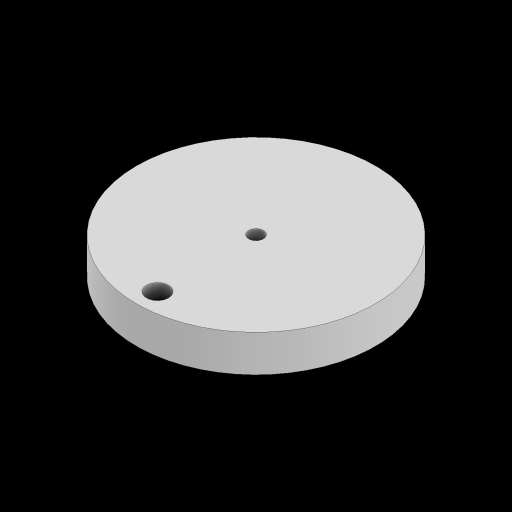
# Autodesk Inventor part: SC-1-02-Circle Arc Cover
Saved by Autodesk Inventor 2023 (Build 270158000, 158)
## iProperties
Created: 2022-12-08
Part Number: SC-1-02-Circle Arc Cover
Material: Generic
Document SubType Name: Modeling
Designer: annah
Density: 1 g/cm^3
Appearance: Default
Author: annah
Autodesk Inventor part; units mm, degrees
ref_plane "YZ Plane" through (0, 0, 0) normal (1, 0, 0) x (0, 1, 0)
ref_plane "XZ Plane" through (0, 0, 0) normal (0, 1, 0) x (-1, 0, 0)
ref_plane "XY Plane" through (0, 0, 0) normal (0, 0, 1) x (1, 0, 0)
sketch "Sketch1" plane through (0, 0, 0) normal (0, 1, 0) x (-1, 0, 0)
  line L0 (0, 0) -> (18.5658, -69.2885)
  circle A0 centre (25.8819, -96.5926) radius 5
  arc A1 (24.729, -72.9816) -> (15.0747, -75.5678) centre (19.8599, -74.1181) ccw
  line L1 (30.6777, -95.1782) -> (24.6448, -72.6673)
  line L2 (21.0523, -97.8867) -> (14.9907, -75.2542)
  circle A2 centre (0, -103.5276) radius 11.6229
  line L3 (21.0523, -97.8867) -> (25.8819, -96.5926)
  arc A3 (-25.8819, -96.5926) -> (26.7197, -101.5219) centre (0, -103.5276) ccw
  circle A4 centre (0, -103.5276) radius 39.9
  arc A5 (57.9067, -50.8394) -> (50.8389, -57.9063) centre (54.2582, -54.2582) ccw
  line L4 (67.1751, -74.2462) -> (50.6094, -57.6767)
  line L5 (74.1567, -67.0879) -> (57.6767, -50.6094)
  circle A6 centre (70.7107, -70.7107) radius 5
  circle A7 centre (51.7638, -89.6575) radius 11.6229
  arc A8 (75.5684, -15.0748) -> (72.9809, -24.7289) centre (74.1181, -19.8599) ccw
  line L6 (95.2985, -30.7115) -> (72.6673, -24.6448)
  line L7 (97.7655, -21.0214) -> (75.2542, -14.9907)
  circle A9 centre (96.5926, -25.8819) radius 5
  circle A10 centre (89.6575, -51.7638) radius 11.6229
  arc A11 (72.9816, 24.729) -> (75.5678, 15.0747) centre (74.1181, 19.8599) ccw
  line L8 (97.8867, 21.0523) -> (75.2542, 14.9907)
  line L9 (95.1782, 30.6777) -> (72.6673, 24.6448)
  circle A12 centre (96.5926, 25.8819) radius 5
  circle A13 centre (103.5276, 0) radius 11.6229
  arc A14 (50.8394, 57.9067) -> (57.9063, 50.8389) centre (54.2582, 54.2582) ccw
  line L10 (74.2462, 67.1751) -> (57.6767, 50.6094)
  line L11 (67.0879, 74.1567) -> (50.6094, 57.6767)
  circle A15 centre (70.7107, 70.7107) radius 5
  circle A16 centre (89.6575, 51.7638) radius 11.6229
  arc A17 (15.0748, 75.5684) -> (24.7289, 72.9809) centre (19.8599, 74.1181) ccw
  line L12 (30.7115, 95.2985) -> (24.6448, 72.6673)
  line L13 (21.0214, 97.7655) -> (14.9907, 75.2542)
  circle A18 centre (25.8819, 96.5926) radius 5
  circle A19 centre (51.7638, 89.6575) radius 11.6229
  arc A20 (-24.729, 72.9816) -> (-15.0747, 75.5678) centre (-19.8599, 74.1181) ccw
  line L14 (-21.0523, 97.8867) -> (-14.9907, 75.2542)
  line L15 (-30.6777, 95.1782) -> (-24.6448, 72.6673)
  circle A21 centre (-25.8819, 96.5926) radius 5
  circle A22 centre (0, 103.5276) radius 11.6229
  arc A23 (-57.9067, 50.8394) -> (-50.8389, 57.9063) centre (-54.2582, 54.2582) ccw
  line L16 (-67.1751, 74.2462) -> (-50.6094, 57.6767)
  line L17 (-74.1567, 67.0879) -> (-57.6767, 50.6094)
  circle A24 centre (-70.7107, 70.7107) radius 5
  circle A25 centre (-51.7638, 89.6575) radius 11.6229
  arc A26 (-75.5684, 15.0748) -> (-72.9809, 24.7289) centre (-74.1181, 19.8599) ccw
  line L18 (-95.2985, 30.7115) -> (-72.6673, 24.6448)
  line L19 (-97.7655, 21.0214) -> (-75.2542, 14.9907)
  circle A27 centre (-96.5926, 25.8819) radius 5
  circle A28 centre (-89.6575, 51.7638) radius 11.6229
  arc A29 (-72.9816, -24.729) -> (-75.5678, -15.0747) centre (-74.1181, -19.8599) ccw
  line L20 (-97.8867, -21.0523) -> (-75.2542, -14.9907)
  line L21 (-95.1782, -30.6777) -> (-72.6673, -24.6448)
  circle A30 centre (-96.5926, -25.8819) radius 5
  circle A31 centre (-103.5276, 0) radius 11.6229
  arc A32 (-50.8394, -57.9067) -> (-57.9063, -50.8389) centre (-54.2582, -54.2582) ccw
  line L22 (-74.2462, -67.1751) -> (-57.6767, -50.6094)
  line L23 (-67.0879, -74.1567) -> (-50.6094, -57.6767)
  circle A33 centre (-70.7107, -70.7107) radius 5
  circle A34 centre (-89.6575, -51.7638) radius 11.6229
  arc A35 (-15.0748, -75.5684) -> (-24.7289, -72.9809) centre (-19.8599, -74.1181) ccw
  line L24 (-30.7115, -95.2985) -> (-24.6448, -72.6673)
  line L25 (-21.0214, -97.7655) -> (-14.9907, -75.2542)
  circle A36 centre (-25.8819, -96.5926) radius 5
  circle A37 centre (-51.7638, -89.6575) radius 11.6229
  circle A38 centre (0, 0) radius 5
  circle A39 centre (0, -103.5276) radius 2
  circle A40 centre (0, -76.7327) radius 5
  circle A41 centre (0, -103.5276) radius 32.5
  circle A42 centre (0, -76.7327) radius 3
  circle A43 centre (0, -103.5276) radius 2
  arc A44 (24.6448, -72.6673) -> (-14.9907, -75.2542) centre (0, 0) ccw
  arc A45 (-4.9973, -76.5698) -> (4.9973, -76.5698) centre (0, 0) ccw
  line L26 (0, 0) -> (0, -63.6276)
  line L27 (0, -71.0276) -> (0, -103.5276)
  arc A46 (21.0199, -97.7659) -> (21.0214, -97.7655) centre (0, 0) ccw
  arc A47 (30.6777, -95.1782) -> (-21.0214, -97.7655) centre (0, 0) ccw
  point P0 (0, 0)
  point P1 (0, 0)
  point P2 (50.7227, -50.7227)
  point P3 (73.9009, -74.5607)
  point P4 (69.2885, -18.5658)
  point P5 (101.2804, -27.621)
  point P6 (69.2885, 18.5658)
  point P7 (101.5219, 26.7197)
  point P8 (50.7227, 50.7227)
  point P9 (74.5607, 73.9009)
  point P10 (18.5658, 69.2885)
  point P11 (27.621, 101.2804)
  point P12 (-18.5658, 69.2885)
  point P13 (-26.7197, 101.5219)
  point P14 (-50.7227, 50.7227)
  point P15 (-73.9009, 74.5607)
  point P16 (-69.2885, 18.5658)
  point P17 (-101.2804, 27.621)
  point P18 (-69.2885, -18.5658)
  point P19 (-101.5219, -26.7197)
  point P20 (-50.7227, -50.7227)
  point P21 (-74.5607, -73.9009)
  point P22 (-18.5658, -69.2885)
  point P23 (-27.621, -101.2804)
  point P24 (40.2917, -91.5236)
  point P25 (59.1159, -80.6555)
  point P26 (67.0867, -74.1578)
  point P27 (74.1567, -67.0879)
  point P28 (80.6555, -59.1159)
  point P29 (91.5236, -40.2917)
  point P30 (95.1777, -30.6791)
  point P31 (97.7655, -21.0214)
  point P32 (99.4077, -10.8682)
  point P33 (99.4077, 10.8682)
  point P34 (97.7659, 21.0199)
  point P35 (95.1782, 30.6777)
  point P36 (91.5236, 40.2917)
  point P37 (80.6555, 59.1159)
  point P38 (74.1578, 67.0867)
  point P39 (67.0879, 74.1567)
  point P40 (59.1159, 80.6555)
  point P41 (40.2917, 91.5236)
  point P42 (30.6791, 95.1777)
  point P43 (21.0214, 97.7655)
  point P44 (10.8682, 99.4077)
  point P45 (-10.8682, 99.4077)
  point P46 (-21.0199, 97.7659)
  point P47 (-30.6777, 95.1782)
  point P48 (-40.2917, 91.5236)
  point P49 (-59.1159, 80.6555)
  point P50 (-67.0867, 74.1578)
  point P51 (-74.1567, 67.0879)
  point P52 (-80.6555, 59.1159)
  point P53 (-91.5236, 40.2917)
  point P54 (-95.1777, 30.6791)
  point P55 (-97.7655, 21.0214)
  point P56 (-99.4077, 10.8682)
  point P57 (-99.4077, -10.8682)
  point P58 (-97.7659, -21.0199)
  point P59 (-95.1782, -30.6777)
  point P60 (-91.5236, -40.2917)
  point P61 (-80.6555, -59.1159)
  point P62 (-74.1578, -67.0867)
  point P63 (-67.0879, -74.1567)
  point P64 (-59.1159, -80.6555)
  point P65 (-40.2917, -91.5236)
  point P66 (-30.6791, -95.1777)
  point P67 (-21.0214, -97.7655)
  point P68 (-10.8682, -99.4077)
  point P69 (10.8682, -99.4077)
  point P70 (-10.8682, -99.4077)
  point P71 (10.8682, -99.4077)
  dimension "d6" = 79.8
  dimension "d11" = 65
  dimension "d4" = 10
  dimension "d5" = 10
  dimension "d7" = 360
  dimension "d8" = 10
  dimension "d9" = 4
  dimension "d10" = 10
  dimension "d12" = 6
  constraints: 111 point on circle, 56 end point, 46 centre point, 27 point on line, 11 coincident, 2 vertical, 2 vertical alignment, 1 concentric, 197 other
  measures "d4" diameter of A0
  measures "d5" diameter of A1
  measures "d8" diameter of A38
  measures "d9" diameter of A39
  measures "d10" diameter of A40
  measures "d12" diameter of A42
extrude "Extrusion1" add sketch "Sketch1" along normal blind 10 contours A41 L1 A0 L2 A1 | A1 L2 A46 A2 L27 A40 A41 | A41 L27 A40 A2 A46 L25 A35 | A35 A44 A41 | L2 A1 | A41 A46 L1 | A35 L25 A36 L24 A41 A44 | A46 A41 L24 A36 A3 A0 | A46 A0 | A0 L3 A46 | L27 A42 A45 A40 | A40 A45 A42 L27 | L24 A46 A41 | A46 L3 A0 | A0 A3 A36 A46 A2 | A40 L27 A42 A45 | A45 A42 L27 A40 | A46 A36 | A36 A3 A46 | A46 A3 A36 L24 | A46 L27 A2 | A2 A46 | A2 L27 A46
body "Solid1"
